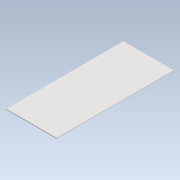
# Autodesk Inventor part: piso
Saved by Autodesk Inventor 2021 (Build 250183000, 183)
## iProperties
Created: 2021-08-22
Part Number: piso
Material: Generic
Document SubType Name: Modeling
Designer: Andrés Holguín
Density: 1 g/cm^3
Appearance: Default
Author: Andrés Holguín
Autodesk Inventor part; units mm, degrees
ref_plane "YZ Plane" through (0, 0, 0) normal (1, 0, 0) x (0, 1, 0)
ref_plane "XZ Plane" through (0, 0, 0) normal (0, 1, 0) x (-1, 0, 0)
ref_plane "XY Plane" through (0, 0, 0) normal (0, 0, 1) x (1, 0, 0)
sketch "Sketch1" plane through (0, 0, 0) normal (0, 1, 0) x (-1, 0, 0)
  line L0 (1278.4823, -2030.2374) -> (-221.5177, -2030.2374)
  line L1 (-221.5177, -2030.2374) -> (-221.5177, 1469.7626)
  line L2 (-221.5177, 1469.7626) -> (1278.4823, 1469.7626)
  line L3 (1278.4823, 1469.7626) -> (1278.4823, -2030.2374)
  point P0 (0, 0)
  dimension "d0" = 1500
  dimension "d1" = 3500
  constraints: 8 end point, 2 parallel, 1 horizontal, 1 perpendicular
  measures "d0" distance of L1.end L2.end
  measures "d1" distance of L0.end L1.end
extrude "Extrusion1" add sketch "Sketch1" along normal blind 25.4
body "Solid1"
